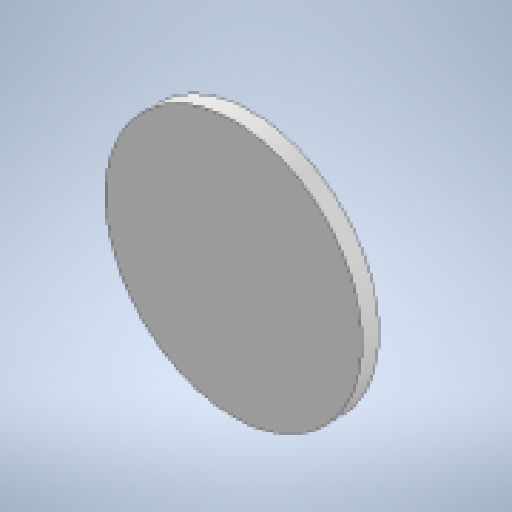
# Autodesk Inventor part: Tapa_Cabeza_Tornillo
Saved by Autodesk Inventor 2024 (Build 280153000, 153)
## iProperties
Created: 2024-07-19
Part Number: Tapa_Cabeza_Tornillo
Material: Genérico
Document SubType Name: Modeling
Designer: sergi
Density: 1 g/cm^3
Appearance: Valor por defecto
Author: sergi
Autodesk Inventor part; units mm, degrees
ref_plane "YZ Plane" through (0, 0, 0) normal (1, 0, 0) x (0, 1, 0)
ref_plane "XZ Plane" through (0, 0, 0) normal (0, 1, 0) x (-1, 0, 0)
ref_plane "XY Plane" through (0, 0, 0) normal (0, 0, 1) x (1, 0, 0)
sketch "Boceto1" plane through (0, 0, 0) normal (0, 0, 1) x (1, 0, 0)
  line L0 (-3.4064, 0) -> (-1.7032, 2.95) projected
  line L1 (-1.7032, 2.95) -> (1.7032, 2.95) projected
  line L2 (1.7032, 2.95) -> (3.4064, 0) projected
  line L3 (3.4064, 0) -> (1.7032, -2.95) projected
  line L4 (1.7032, -2.95) -> (-1.7032, -2.95) projected
  line L5 (-1.7032, -2.95) -> (-3.4064, 0) projected
  circle A0 centre (0, 0) radius 7.5 projected
extrude "Extrusión1" add sketch "Boceto1" along normal blind 1 contours L0 L1 L2 L3 L4 L5 | A0
sketch "Boceto2" plane through (0, 0, 0) normal (0, 0, -1) x (-1, 0, 0)
  circle A0 centre (0, 0) radius 7.5 projected
  circle A1 centre (0, 0) radius 1.5 projected
  line L0 (1.7032, -2.95) -> (3.4064, 0) projected
  line L1 (3.4064, 0) -> (1.7032, 2.95) projected
  line L2 (1.7032, 2.95) -> (-1.7032, 2.95) projected
  line L3 (-1.7032, 2.95) -> (-3.4064, 0) projected
  line L4 (-3.4064, 0) -> (-1.7032, -2.95) projected
  line L5 (-1.7032, -2.95) -> (1.7032, -2.95) projected
  line L6 (-1.5588, -2.7) -> (-3.1177, 0)
  line L7 (-3.1177, 0) -> (-1.5588, 2.7)
  line L8 (-1.5588, 2.7) -> (1.5588, 2.7)
  line L9 (1.5588, 2.7) -> (3.1177, 0)
  line L10 (3.1177, 0) -> (1.5588, -2.7)
  line L11 (1.5588, -2.7) -> (-1.5588, -2.7)
  dimension "d2" = 0.25
  constraints: 12 end point, 5 other
  measures "d2" distance between parallel lines of L4 L6
extrude "Extrusión2" add sketch "Boceto2" along normal blind 1.6 contours A1 | L6 L7 L8 L9 L10 L11
